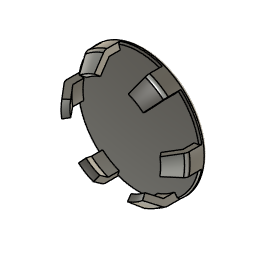
Reflektor v1 (Autodesk Fusion 360 design; units mm, degrees)
Autodesk Fusion 360 part; units mm, degrees
sketch "Skizze1" plane through (0, 0, 0) normal (0, 0, 1) x (1, 0, 0)
  circle A0 centre (0, 0) radius 20
  line L0 (0, 50) -> (0, -36.4171) construction
  line L1 (-20, 23) -> (20, 23)
  line L2 (20, 23) -> (20, 16.6992)
  line L3 (20, 16.6992) -> (16.0259, 11.9654)
  line L4 (-20, 23) -> (-20, 16.6992)
  line L5 (-20, 16.6992) -> (-16.0259, 11.9654)
  line L6 (-16.0259, 11.9654) -> (16.0259, 11.9654) construction
  line L7 (-18, 21) -> (18, 21)
  line L8 (18, 21) -> (18, 17.4274)
  line L9 (18, 17.4274) -> (14.7285, 13.5304)
  line L10 (-18, 21) -> (-18, 17.4274)
  line L11 (-18, 17.4274) -> (-14.7285, 13.5304)
  line L12 (0, 23) -> (0, 21)
  point P0 (0, 20)
  dimension "d1" = 40
  dimension "d2" = 40
  dimension "d3" = 3
  dimension "d4" = 2
  dimension "d5" = 2
  dimension "d6" = 2
  dimension "d7" = 2
  dimension "d8" = 2
  constraint coincident A0.centre origin
  constraint vertical L0
  constraint perpendicular L0 L1
  constraint perpendicular L1 L2
  constraint coincident A0 L3.end
  constraint perpendicular L1 L4
  constraint coincident A0 L5.end
  constraint symmetric L0 L1.start L1.end
  constraint symmetric L0 L2.end L4.end
  constraint coincident A0.centre L0
  constraint coincident A0 P0
  constraint coincident L0 P0
  constraint horizontal L6
  constraint parallel L1 L7
  constraint perpendicular L7 L8
  constraint coincident A0 L9.end
  constraint coincident A0 L11.end
  constraint parallel L3 L9
  constraint parallel L5 L11
  constraint vertical L10
  constraint midpoint L1 L12.start
  constraint midpoint L7 L12.end
  measures "d1" diameter of A0
  measures "d2" distance of L1.start L1.end
  measures "d3" distance of L1 P0
  measures "d4" distance of L1 L7
  measures "d5" distance of L4 L10
  measures "d6" distance of L2 L8
  measures "d7" distance of L3 L9
  measures "d8" distance of L5 L11
revolve "Drehen1" add sketch "Skizze1" angle 360 about axis through (0, 50, 0) along (0, -1, 0) contours A0 L1 L4 L5 L7 L10 L11 L12
sketch "Skizze2" plane through (0, 21, 0) normal (0, -1, 0) x (1, 0, 0)
  circle A0 centre (0, 0) radius 18
  circle A1 centre (0, 0) radius 20.5
  line L0 (0, 0) -> (7.1898, 19.1978)
  line L1 (0, 0) -> (13.3222, 15.581)
  line L2 (0, 0) -> (17.8478, 10.0849)
  line L3 (0, 0) -> (20.2207, 3.3724)
  line L4 (0, 0) -> (20.1547, -3.7469)
  line L5 (0, 0) -> (0.1901, 20.4991)
  line L6 (0, 0) -> (-6.8324, 19.3279)
  line L7 (0, 0) -> (-13.0309, 15.8255)
  line L8 (0, 0) -> (-17.6577, 10.4142)
  line L9 (0, 0) -> (-20.1547, 3.7469)
  line L10 (0, 0) -> (-20.2207, -3.3724)
  line L11 (0, 0) -> (-17.8478, -10.0849)
  line L12 (0, 0) -> (-13.3222, -15.581)
  line L13 (0, 0) -> (17.6577, -10.4142)
  line L14 (0, 0) -> (13.0309, -15.8255)
  line L15 (0, 0) -> (6.8324, -19.3279)
  line L16 (0, 0) -> (-7.1898, -19.1978)
  line L17 (0, 0) -> (-0.1901, -20.4991)
  dimension "d10" = 41
  dimension "d12" = 20
  dimension "d13" = 20
  dimension "d14" = 20
  dimension "d15" = 20
  dimension "d16" = 20
  dimension "d17" = 20
  dimension "d18" = 20
  dimension "d19" = 20
  dimension "d20" = 20
  dimension "d21" = 20
  dimension "d22" = 20
  dimension "d23" = 20
  dimension "d24" = 20
  dimension "d25" = 20
  dimension "d26" = 20
  dimension "d27" = 20
  dimension "d28" = 20
  constraint coincident A0.centre A1.centre
  constraint coincident A1 L0.end
  constraint coincident A1 L1.end
  constraint coincident A1 L2.end
  constraint coincident A1 L3.end
  constraint coincident A1 L4.end
  constraint coincident A1 L5.end
  constraint coincident A1 L6.end
  constraint coincident A1 L7.end
  constraint coincident A1 L8.end
  constraint coincident A1 L9.end
  constraint coincident A1 L10.end
  constraint coincident A1 L11.end
  constraint coincident A1 L12.end
  constraint coincident A1 L13.end
  constraint coincident A1 L14.end
  constraint coincident A1 L15.end
  constraint coincident A1 L16.end
  constraint coincident A1 L17.end
  measures "d10" diameter of A1
  measures "d12" angle of L0 L5
  measures "d13" angle of L0 L1
  measures "d14" angle of L1 L2
  measures "d15" angle of L2 L3
  measures "d16" angle of L3 L4
  measures "d17" angle of L5 L6
  measures "d18" angle of L6 L7
  measures "d19" angle of L7 L8
  measures "d20" angle of L8 L9
  measures "d21" angle of L9 L10
  measures "d22" angle of L10 L11
  measures "d23" angle of L11 L12
  measures "d24" angle of L12 L16
  measures "d25" angle of L4 L13
  measures "d26" angle of L13 L14
  measures "d27" angle of L14 L15
  measures "d28" angle of L16 L17
extrude "Extrusion1" cut sketch "Skizze2" along normal blind 20 contours A0 L2 L3 | A0 A1 L2 L3 | A0 A1 L4 L13 | A0 L4 L13 | A0 L1 L2 | A0 A1 L1 L2 | A0 L0 L5 | A0 L5 L6 | A0 L7 L8 | A0 L8 L9 | A0 L10 L11 | A0 L11 L12 | A0 L13 L14 | A0 L16 L17 | A0 L15 L17 | A0 A1 L13 L14 | A0 A1 L0 L5 | A0 A1 L5 L6 | A0 A1 L7 L8 | A0 A1 L8 L9 | A0 A1 L10 L11 | A0 A1 L11 L12 | A0 A1 L15 L17 | A0 A1 L16 L17
fillet "Abrundung1" radius 2 6 edges at (-10.1602, 16.6992, -17.227) (9.8389, 16.6992, -17.4125) (19.9991, 16.6992, -0.1855) (-19.9991, 16.6992, 0.1855) (-9.8389, 16.6992, 17.4125) (10.1602, 16.6992, 17.227)
chamfer "Fase1" distance 0.5 angle 45 6 edges at (17.227, 21, -10.1602) (-0.1855, 21, -19.9991) (17.4125, 21, 9.8389) (0.1855, 21, 19.9991) (-17.227, 21, 10.1602) (-17.4125, 21, -9.8389)
fillet "Abrundung2" radius 1 1 edges at (-18.6465, 23, 7.2323)
